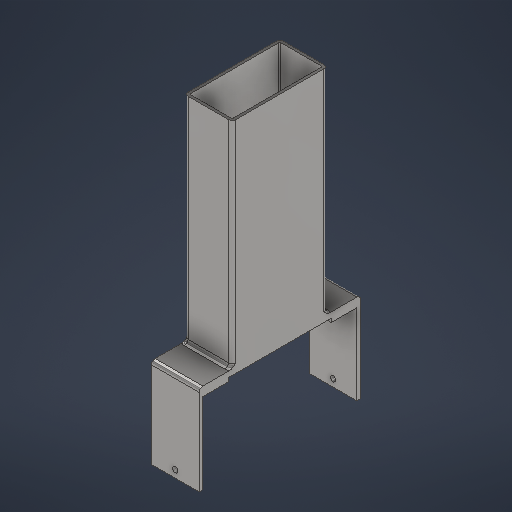
# Autodesk Inventor part: SACMI DPA CARDBOARD CONVEYOR SUPPORT
Saved by Autodesk Inventor 2025 (Build 290162000, 162)
## iProperties
Created: 2024-05-26
Part Number: SACMI DPA CARDBOARD CONVEYOR SUPPORT
Material: Generic
Document SubType Name: Modeling
Designer: zulet
Density: 1 g/cm^3
Appearance: Steel - Polished
Author: zulet
Autodesk Inventor part; units mm, degrees
ref_plane "YZ Plane" through (0, 0, 0) normal (1, 0, 0) x (0, 1, 0)
ref_plane "XZ Plane" through (0, 0, 0) normal (0, 1, 0) x (-1, 0, 0)
ref_plane "XY Plane" through (0, 0, 0) normal (0, 0, 1) x (1, 0, 0)
sketch "Sketch1" plane through (0, 0, 0) normal (1, 0, 0) x (0, 1, 0)
  line L0 (0, 210) -> (220, 210)
  line L1 (220, 210) -> (220, 140)
  line L2 (220, 140) -> (230, 140)
  line L3 (230, 140) -> (230, 0)
  line L4 (0, 210) -> (0, 220)
  line L5 (0, 220) -> (245, 220)
  line L6 (245, 220) -> (245, 130)
  line L7 (245, 130) -> (829, 130)
  line L8 (829, 130) -> (829, 0)
  line L9 (829, 0) -> (230, 0) construction
  line L10 (-165.8, 0) -> (994.8, 0) construction
  line L11 (0, -308) -> (0, 308) construction
  line L12 (0, -210) -> (220, -210)
  line L13 (220, -210) -> (220, -140)
  line L14 (220, -140) -> (230, -140)
  line L15 (230, -140) -> (230, 0)
  line L16 (0, -210) -> (0, -220)
  line L17 (0, -220) -> (245, -220)
  line L18 (245, -220) -> (245, -130)
  line L19 (245, -130) -> (829, -130)
  line L20 (829, -130) -> (829, 0)
  point P0 (0, 0)
  dimension "d0" = 420
  dimension "d1" = 829
  dimension "d2" = 230
  dimension "d3" = 10
  dimension "d4" = 140
  dimension "d5" = 10
  dimension "d6" = 25
  dimension "d18" = 260
  constraints: 38 end point, 8 symmetric about line, 7 perpendicular, 2 collinear, 2 vertical, 1 horizontal
  measures "d0" distance between parallel lines of L12 L0
  measures "d1" distance between parallel lines of L4 L8
  measures "d2" distance between parallel lines of L4 L3
  measures "d3" distance between parallel lines of L3 L1
  measures "d4" distance between parallel lines of L9 L2
  measures "d5" distance between parallel lines of L5 L0
  measures "d6" distance between parallel lines of L1 L6
  measures "d18" distance between parallel lines of L19 L7
extrude "Extrusion1" add sketch "Sketch1" along normal blind 130
sketch "Sketch2" plane through (0, 0, -220) normal (0, 0, -1) x (-1, 0, 0)
  line L0 (0, 0) -> (-130, 0) construction
  line L1 (-65, 0) -> (-65, 245) construction
  line L2 (0, 245) -> (-130, 245) construction
  circle A0 centre (-65, 20) radius 7.5
  dimension "d10" = 15
  dimension "d11" = 20
  constraints: 2 end point, 2 midpoint, 1 centre point, 1 point on line
  measures "d10" diameter of A0
  measures "d11" distance from line of L0 A0.centre
extrude "Extrusion2" cut sketch "Sketch2" against normal through all
fillet "Fillet1" radius 10 6 edges at (130, 537, 130) (130, 537, -130) (0, 537, -130) (0, 537, 130) (65, 245, 220) (65, 245, -220)
sketch "Sketch3" plane through (0, 829, 120) normal (0, 1, 0) x (1, 0, 0)
  arc A0 (0, 0) -> (10, -10) centre (10, 0) ccw projected
  line L0 (10, -10) -> (120, -10) projected
  arc A1 (120, -10) -> (130, 0) centre (120, 0) ccw projected
  line L1 (130, 240) -> (130, 0) projected
  arc A2 (130, 240) -> (120, 250) centre (120, 240) ccw projected
  line L2 (10, 250) -> (120, 250) projected
  arc A3 (10, 250) -> (0, 240) centre (10, 240) ccw projected
  line L3 (0, 240) -> (0, 0) projected
  arc A4 (7, 0) -> (10, -3) centre (10, 0) ccw
  line L4 (10, -3) -> (120, -3)
  arc A5 (120, -3) -> (123, 0) centre (120, 0) ccw
  line L5 (123, 0) -> (123, 240)
  arc A6 (123, 240) -> (120, 243) centre (120, 240) ccw
  line L6 (120, 243) -> (10, 243)
  arc A7 (10, 243) -> (7, 240) centre (10, 240) ccw
  line L7 (7, 240) -> (7, 0)
  point P0 (0, 120)
  dimension "d15" = 7
  constraints: 8 end point, 8 point on circle, 4 centre point, 7 other
  measures "d15" distance between parallel lines of L3 L7
extrude "Extrusion3" cut sketch "Sketch3" against normal up to surface (584 mm away) contours L7 A7 L6 A6 L5 A5 L4 A4
fillet "Fillet2" radius 10 6 edges at (127.0711, 245, 127.0711) (2.9289, 245, 127.0711) (65, 245, 130) (127.0711, 245, -127.0711) (2.9289, 245, -127.0711) (65, 245, -130)
body "Solid1"
